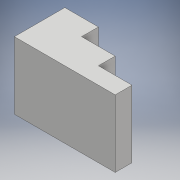
# Autodesk Inventor part: 46
Saved by Autodesk Inventor 2017 (Build 210142000, 142)
## iProperties
Part Number: 46
Material: 一般
Document SubType Name: Modeling
Designer: Brian
Density: 1 g/cm^3
Appearance: 預設
Author: Brian
Autodesk Inventor part; units mm, degrees
ref_plane "YZ Plane" through (0, 0, 0) normal (1, 0, 0) x (0, 1, 0)
ref_plane "XZ Plane" through (0, 0, 0) normal (0, 1, 0) x (-1, 0, 0)
ref_plane "XY Plane" through (0, 0, 0) normal (0, 0, 1) x (1, 0, 0)
sketch "草圖1" plane through (0, 0, 0) normal (0, 1, 0) x (-1, 0, 0)
  line L0 (0, 0) -> (-60, 0)
  line L1 (-60, 0) -> (-60, -40)
  line L2 (-60, -40) -> (0, -40)
  line L3 (0, -40) -> (0, 0)
  dimension "d0" = 60
  dimension "d1" = 40
  constraints: 8 end point, 2 parallel, 1 horizontal, 1 perpendicular
  measures "d0" distance of L1.end L2.end
  measures "d1" distance of L0.end L1.end
extrude "擠出1" add sketch "草圖1" along normal blind 10
sketch "草圖2" plane through (0, 10, 0) normal (0, 1, 0) x (1, 0, 0)
  line L0 (0, 40) -> (0, 0) projected
  line L1 (0, 0) -> (60, 0) projected
  line L2 (0, 40) -> (20, 40)
  line L3 (20, 40) -> (20, 0)
  line L4 (20, 0) -> (0, 0)
  line L5 (0, 0) -> (0, 40)
  dimension "d4" = 20
  constraints: 8 end point, 2 parallel, 1 horizontal, 1 perpendicular, 1 point on line
  measures "d4" distance between parallel lines of L0 L3
extrude "擠出2" add sketch "草圖2" along normal blind 20
sketch "草圖3" plane through (0, 10, 0) normal (0, 1, 0) x (1, 0, 0)
  line L0 (20, 0) -> (20, 40) projected
  line L1 (20, 40) -> (40, 40)
  line L2 (40, 40) -> (40, 30)
  line L3 (40, 30) -> (20, 30)
  line L4 (20, 30) -> (20, 40)
  line L5 (0, 0) -> (60, 0) projected
  line L6 (20, 0) -> (40, 0)
  line L7 (40, 0) -> (40, 10)
  line L8 (40, 10) -> (20, 10)
  line L9 (20, 10) -> (20, 0)
  dimension "d7" = 20
  dimension "d8" = 10
  dimension "d9" = 10
  constraints: 16 end point, 4 parallel, 3 point on line, 2 horizontal, 2 perpendicular
  measures "d7" distance of L7.end L8.end
  measures "d8" distance of L1.end L2.end
  measures "d9" distance of L6.end L7.end
extrude "擠出3" add sketch "草圖3" along normal blind 10
